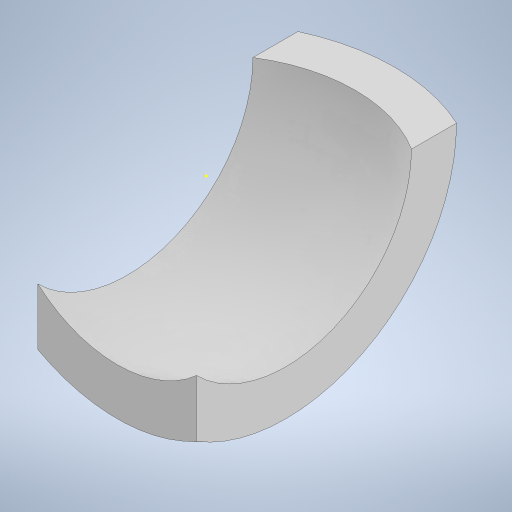
# Autodesk Inventor part: tail12.16
Saved by Autodesk Inventor 2023 (Build 270158000, 158)
## iProperties
Created: 2022-12-16
Part Number: tail12.16
Material: 一般
Document SubType Name: Modeling
Designer: ellie
Density: 1 g/cm^3
Appearance: 既定
Author: ellie
Autodesk Inventor part; units mm, degrees
ref_plane "YZ Plane" through (0, 0, 0) normal (1, 0, 0) x (0, 1, 0)
ref_plane "XZ Plane" through (0, 0, 0) normal (0, 1, 0) x (-1, 0, 0)
ref_plane "XY Plane" through (0, 0, 0) normal (0, 0, 1) x (1, 0, 0)
sketch "スケッチ1" plane through (0, 0, 0) normal (0, 1, 0) x (-1, 0, 0)
  circle A0 centre (0, 0) radius 37.5
  circle A1 centre (0, 0) radius 47.5
  line L0 (0, -47.5) -> (0, 47.5)
  point P0 (0, -37.5)
  point P1 (0, 37.5)
  dimension "d0" = 75
  dimension "d1" = 95
  dimension "d2" = 95
  constraints: 2 centre point, 2 coincident, 2 end point, 2 point on circle, 1 vertical
  measures "d0" diameter of A0
  measures "d1" diameter of A1
  measures "d2" distance of L0.start L0.end
sketch "スケッチ2" plane through (0, 0, 0) normal (0, 1, 0) x (-1, 0, 0)
  point P0 (0, 0)
revolve "回転1" add sketch "スケッチ1" angle 180 about axis through (0, 0, -47.5) along (0, 0, 1) picked at (43.8624, 3.0889) contours A0 L0 A1
sketch "スケッチ3" plane through (0, 0, 0) normal (0, 1, 0) x (1, 0, 0)
  line L0 (20, -47.5) -> (-20, -47.5)
  line L1 (-20, -47.5) -> (-20, 47.5)
  line L2 (-20, 47.5) -> (20, 47.5)
  line L3 (20, 47.5) -> (20, -47.5)
  circle A0 centre (0, 0) radius 47.5 projected
  line L4 (0, -47.5) -> (0, 47.5)
  point P0 (-20, 43.0842)
  point P1 (-20, -43.0842)
  point P2 (20, 43.0842)
  point P3 (20, -43.0842)
  dimension "d4" = 95
  dimension "d5" = 40
  constraints: 10 end point, 2 parallel, 2 point on circle, 2 tangent, 1 horizontal, 1 perpendicular, 1 vertical, 1 other
  measures "d4" distance of L4.start L4.end
  measures "d5" distance of L0.start L0.end
extrude "押し出し1" cut sketch "スケッチ3" against normal blind 100 contours L3 A0 | A0 L1
sketch "スケッチ4" plane through (0, 0, 0) normal (0, 1, 0) x (1, 0, 0)
  line L0 (-20, 47.5) -> (20, 47.5)
  line L1 (20, 47.5) -> (20, -22.5)
  line L2 (20, -22.5) -> (-20, -22.5)
  line L3 (-20, -22.5) -> (-20, 47.5)
  arc A0 (20, 43.0842) -> (-20, 43.0842) centre (0, 0) ccw projected
  line L4 (-20, 43.0842) -> (-20, 31.7214) projected
  line L5 (20, 31.7214) -> (20, 43.0842) projected
  line L6 (20, 43.0842) -> (20, 31.7214) projected
  arc A1 (20, 31.7214) -> (-20, 31.7214) centre (0, 0) ccw projected
  line L7 (-20, 31.7214) -> (-20, 43.0842) projected
  arc A2 (20, 43.0842) -> (-20, 43.0842) centre (0, 0) ccw projected
  line L8 (20, -31.7214) -> (20, -43.0842) projected
  arc A3 (-20, -43.0842) -> (20, -43.0842) centre (0, 0) ccw projected
  line L9 (-20, -43.0842) -> (-20, -31.7214) projected
  arc A4 (-20, -31.7214) -> (20, -31.7214) centre (0, 0) ccw projected
  line L10 (20, 43.0842) -> (20, 31.7214) projected
  arc A5 (20, 31.7214) -> (-20, 31.7214) centre (0, 0) ccw projected
  line L11 (-20, 31.7214) -> (-20, 43.0842) projected
  arc A6 (20, 43.0842) -> (-20, 43.0842) centre (0, 0) ccw projected
  line L12 (20, -31.7214) -> (20, -43.0842) projected
  arc A7 (-20, -43.0842) -> (20, -43.0842) centre (0, 0) ccw projected
  line L13 (-20, -43.0842) -> (-20, -31.7214) projected
  arc A8 (-20, -31.7214) -> (20, -31.7214) centre (0, 0) ccw projected
  line L14 (-20, 31.7214) -> (-20, -31.7214) projected
  arc A9 (-20, -31.7214) -> (20, -31.7214) centre (0, 0) ccw projected
  line L15 (20, -31.7214) -> (20, 31.7214) projected
  arc A10 (20, 31.7214) -> (-20, 31.7214) centre (0, 0) ccw projected
  point P0 (-20, 43.0842)
  point P1 (0, 47.5)
  point P2 (20, 43.0842)
  dimension "d8" = 70
  constraints: 8 end point, 2 collinear, 2 parallel, 1 horizontal, 1 perpendicular, 1 tangent
  measures "d8" distance of L2.end L0.start
extrude "押し出し2" cut sketch "スケッチ4" against normal blind 100 contours L2 L15 A4 L14 | A4 L8 A3 L9
